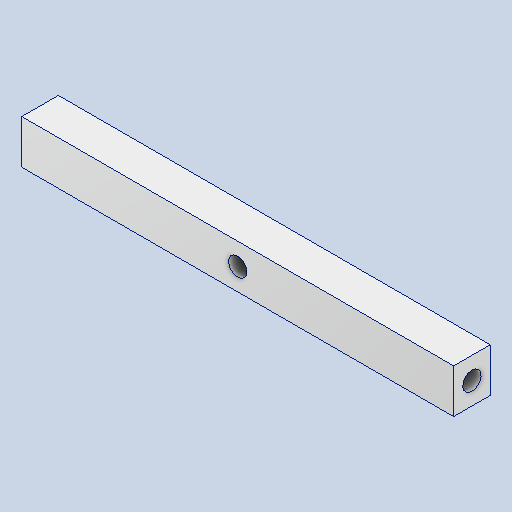
# Autodesk Inventor part: belt_liner_v2_Plate_7
Saved by Autodesk Inventor 2025.2 (Build 292293000, 293)
## iProperties
Created: 2025-01-06
Part Number: belt_liner_v2_Plate_7
Material: アルミニウム 6061
Document SubType Name: Modeling
Designer: haruy
Density: 2.7 g/cm^3
Appearance: アルミニウム - フラット
Author: haruy
Autodesk Inventor part; units mm, degrees
ref_plane "YZ Plane" through (0, 0, 0) normal (1, 0, 0) x (0, 1, 0)
ref_plane "XZ Plane" through (0, 0, 0) normal (0, 1, 0) x (-1, 0, 0)
sketch "スケッチ1" plane through (0, 0, 0) normal (1, 0, 0) x (0, 1, 0)
  line L0 (0, 0) -> (6, 0)
  line L1 (6, 0) -> (6, -5)
  line L2 (6, -5) -> (0, -5)
  line L3 (0, -5) -> (0, 0)
  point P0 (3, -2.5)
  dimension "d0" = 6
  dimension "d1" = 5
  dimension "d2" = 3
  dimension "d3" = 2.5
  constraints: 8 end point, 2 parallel, 1 horizontal, 1 perpendicular
  measures "d0" distance of L1.end L2.end
  measures "d1" distance of L0.end L1.end
  measures "d2" distance from line of point (3, -2.5) L1
  measures "d3" distance from line of point (3, -2.5) L0
extrude "押し出し1" add sketch "スケッチ1" against normal blind 59
ref_plane "作業平面1" through (-29.5, 0, 0) normal (1, 0, 0) x (0, 0, -1)
hole "穴1" at (0, 3, -2.5) direction (-1, 0, 0) diameter 2.5 depth 5 tip angle 118
mirror "ミラー1" about plane through (-29.5, 0, 0) normal (1, 0, 0) of "穴1"
sketch "スケッチ2" plane through (0, 0, 0) normal (0, 0, 1) x (1, 0, 0)
  circle A0 centre (-29.5, 3) radius 1.25
  line L0 (0, 6) -> (-59, 6) projected
  line L1 (0, 6) -> (0, 0) projected
  dimension "d14" = 2.5
  dimension "d15" = 3
  dimension "d16" = 29.5
  constraints: 1 centre point
  measures "d14" diameter of A0
  measures "d15" distance from line of A0.centre L0
  measures "d16" distance from line of A0.centre L1
extrude "押し出し2" cut sketch "スケッチ2" against normal blind 59
